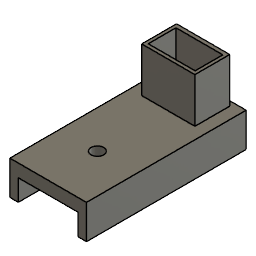
soporte_infrarrojo (Autodesk Fusion 360 design; units mm, degrees)
Autodesk Fusion 360 part; units mm, degrees
note: some values were not read from the file. Set by a fixed rule: which sketch regions a step uses.
sketch "Boceto1" plane through (0, 0, 0) normal (0, 1, 0) x (1, 0, 0)
  line L0 (9, -18.75) -> (-9, -18.75)
  line L1 (-9, -18.75) -> (-9, 18.75)
  line L2 (-9, 18.75) -> (9, 18.75)
  line L3 (9, 18.75) -> (9, -18.75)
  line L4 (9, -18.75) -> (-9, 18.75) construction
  line L5 (-9, -18.75) -> (9, 18.75) construction
  line L6 (5.5, 16.75) -> (-5.5, 16.75)
  line L7 (-5.5, 16.75) -> (-5.5, 10.25)
  line L8 (-5.5, 10.25) -> (5.5, 10.25)
  line L9 (0, -18.75) -> (0, -8.55)
  circle A0 centre (-0.1319, -7.0558) radius 1.5
  line L10 (0, -20) -> (0, 20) construction
  line L11 (6.25, 9.45) -> (-6.25, 9.45)
  line L12 (-6.25, 9.45) -> (-6.25, 17.65)
  line L13 (-6.25, 17.65) -> (6.25, 17.65)
  line L14 (6.25, 17.65) -> (6.25, 9.45)
  line L15 (6.25, 9.45) -> (-6.25, 17.65) construction
  line L16 (-6.25, 9.45) -> (6.25, 17.65) construction
  line L17 (5.5, 16.75) -> (5.5, 10.25)
  point P0 (0, 13.55)
  point P1 (0, 13.55)
  dimension "d1" = 18
  dimension "d2" = 37.5
  dimension "d8" = 2
  dimension "d9" = 6.5
  dimension "d18" = 11
  dimension "d20" = 10.2
  dimension "d21" = 3
  dimension "d26" = 12.5
  dimension "d27" = 8.2
  dimension "d28" = 5.5
  dimension "d29" = 0.75
  dimension "d30" = 0.8
  constraint horizontal L0
  constraint perpendicular L0 L1
  constraint parallel L0 L2
  constraint parallel L1 L3
  constraint coincident L4 origin
  constraint coincident L5 origin
  constraint perpendicular L6 L7
  constraint midpoint L0 L9.start
  constraint perpendicular L0 L9
  constraint coincident L9.end A0
  constraint midpoint L10 origin
  constraint perpendicular L2 L10
  constraint horizontal L11
  constraint perpendicular L11 L12
  constraint parallel L11 L13
  constraint parallel L12 L14
  constraint coincident L15 P1
  constraint coincident L16 P1
  constraint coincident P1 P0
  constraint perpendicular L8 L17
  measures "d1" distance of L1.end L2.end
  measures "d2" distance of L0.end L1.end
  measures "d8" distance of L2 L6
  measures "d9" distance of L6.end L7.end
  measures "d18" distance of L7.end L8.end
  measures "d20" distance of L9.start L9.end
  measures "d21" diameter of A0
  measures "d26" distance of L12.end L13.end
  measures "d27" distance of L11.end L12.end
  measures "d28" distance of L7 L10
  measures "d29" distance of L14 L17
  measures "d30" distance of L8 L11
extrude "Extruir1" add sketch "Boceto1" along normal blind 13.5 contours L11 L12 L13 L14
extrude "Extruir2" add sketch "Boceto1" along normal blind 3 contours L0 L1 L2 L3
sketch "Boceto2" plane through (0, 0, 0) normal (0, -1, 0) x (1, 0, 0)
  circle A0 centre (-0.1319, 7.0558) radius 1.5
  line L0 (-9, -18.75) -> (9, -18.75)
  line L1 (9, -18.75) -> (9, 18.75)
  line L2 (9, 18.75) -> (-9, 18.75)
  line L3 (-9, 18.75) -> (-9, -18.75)
  line L4 (-5.5, -16.75) -> (-5.5, -10.25)
  line L5 (-5.5, -10.25) -> (5.5, -10.25)
  line L6 (5.5, -10.25) -> (5.5, -16.75)
  line L7 (5.5, -16.75) -> (-5.5, -16.75)
  line L8 (-9, 18.75) -> (-7, 18.75)
  line L9 (-7, 18.75) -> (-7, -18.75)
  line L10 (-7, -18.75) -> (-9, -18.75)
  line L11 (-9, -18.75) -> (-9, 18.75)
  line L12 (9, 18.75) -> (7, 18.75)
  line L13 (7, 18.75) -> (7, -18.75)
  line L14 (7, -18.75) -> (9, -18.75)
  line L15 (9, -18.75) -> (9, 18.75)
  dimension "d34" = 2
  dimension "d35" = 2
  constraint horizontal L8
  constraint vertical L9
  constraint horizontal L10
  constraint vertical L11
  constraint coincident L2.end L3.start
  constraint horizontal L12
  constraint vertical L13
  constraint horizontal L14
  constraint vertical L15
  constraint coincident L1.end L2.start
  measures "d34" distance of L2.end L8.end
  measures "d35" distance of L1.end L12.end
extrude "Extruir4" add sketch "Boceto2" along normal blind 5 contours L0 L2 L3 L8 L9 L10 L11 | L0 L1 L2 L12 L13 L14 L15
